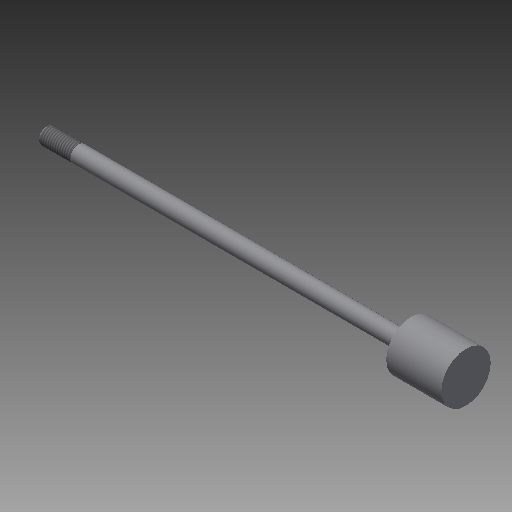
# Autodesk Inventor part: 043.5-DXP0000_rod
Saved by Autodesk Inventor 2019 (Build 230136000, 136)
## iProperties
Category: PARTsolutions
Company: BIMBA
Created: 2019-01-26
Part Number: 043.5-DXP0000_rod
Material: Generic
Catalog Web Link: www.cadenas.de
Description: Standard Air Cylinder_rod-Original Line - Standard Air Cylinders
Vendor: BIMBA
Document SubType Name: Modeling
Designer: psadmin
Manufacturer: BIMBA
Mass: 10.7288 g
Surface Area: 47.1446 cm^2
Volume: 10.7288 cm^3
Density: 1 g/cm^3
Appearance: PSOLRGB-181-181-181
PSOL_IDENT_0: {$CADENAS_DATA\23d-libs\bimba\bimba\bimba_imperial\bimba_full_line\original_line_cylinders\standard_
PSOL_IDENT_1: air_cylinders\rod.prj},327 {VTYP=3D},{NB=043.5-DXP0000_rod},{LINA=043.5-DXP0000_rod},{NN=Standard Ai
PSOL_IDENT_2: r Cylinder_rod},{DATE=21.03.2018 14:31:21},{GEOMDATE=09.11.2017 13:09:15},{VERSION=},{LINEID=50},{WB
PSOL_IDENT_3: VAR=STROKE,ACTING,MNT,DER,NR,BM,CO,M,EE,EEL,K,Q,Y,F,G,T,B,H,SER,SR,NT,W,E,HL,ST,STP,PRC,PB,COLOR1,FC
PSOL_IDENT_4: D,RCD,BCD},{WBNUMERIC=STROKE,EEL,COLOR1,FCD,RCD,BCD}  {NB=043.5-DXP0000_rod},{LINA=043.5-DXP0000_rod
PSOL_IDENT_5: },{KT=DUMMY},{PN=043.5-DXP000},{DASH=-},{BORE=0.75000000},{BOREPN=04},{STROKE=3.500},{STROKEALG=[0.0
PSOL_IDENT_6: 01:50/0.001]},{STROKE1=3.500},{ACTING=D},{ACTINGALG= '' , 'Single Acting' , 'R' , 'Reverse Single Ac
PSOL_IDENT_7: ting' , 'D' , 'Double Acting' },{ACTINGPN=D},{MNT=XP},{MNTALG= '' , 'Front Nose Mounting' , 'P' , 'R
PSOL_IDENT_8: ear Pivot Mounting' , 'XP' , 'Double End or Pivot Mounting' , 'X' , 'Double End Mounting' , 'BF' , '
PSOL_IDENT_9: Front Block Mounting' , 'BR' , 'Rear Block Mounting for Vertical Positioning' , 'BFT' , 'Front Block
PSOL_IDENT_10: Trunnion Mounting' , 'BRT' , 'Rear Block Trunnion Mounting' },{TYPE=},{MNTPN=XP},{DER=},{DERALG= ''
PSOL_IDENT_11: , 'N/A' },{NR=},{NRALG= '' , 'N/A' },{NRPN=},{BM=},{BMALG= '' , 'N/A' },{BMPN=},{CO=},{COALG= '' , '
PSOL_IDENT_12: N/A' },{M=},{MALG= '', 'Without Magnet', 'M', 'With Magnet' },{EE=},{EEL=0},{EEMAX=46},{EEALG= '', '
PSOL_IDENT_13: Without Extra Extension', 'EE', 'With Extra Extension' },{EELALG=0},{EEPN=},{EEPN1=0.000},{K=},{KALG=
PSOL_IDENT_14: '', 'Standard' , 'K' , 'Ports Rotated 90deg' },{KPN=},{Q=},{QALG= '' , 'Without Side Ported Rear He
PSOL_IDENT_15: ad' , 'Q' , 'With Side Ported Rear Head' },{QPN=},{Y=},{YALG= '' , 'Without Pivot Bushing' , 'Y' , '
PSOL_IDENT_16: With Pivot Bushing' },{YPN=},{F=},{FALG= '', 'Standard', 'F', 'Molycoated Body' },{FPN=},{G=},{GPN=}
PSOL_IDENT_17: ,{T=},{TALG= '' , 'Standard' , 'N' , 'Low Temperature' , 'V' , 'High Temperature' },{NPN=},{VPN=},{B=
PSOL_IDENT_18: },{BALG= '', 'Without Bumper' , 'B' , 'With Bumper' },{BPN=},{H=},{HALG= '', 'N/A' },{HPN=},{SER=},{
PSOL_IDENT_19: SERALG= '' , 'Without Spring Extend/Return' , 'JS' , 'With Spring Return' , 'JR' , 'With Spring Exte
PSOL_IDENT_20: nd' },{SR=},{SRALG= 'C' , 'Carbon Steel Rod' , 'SR' , '303 Stainless Steel Rod' , '' , '303 Stainles
PSOL_IDENT_21: s Steel Rod1' },{SRPN=},{SRCON=0},{NT=},{NTPN=},{W=},{WALG= '' , 'Without Wiper' , 'W' , 'With Wiper'
PSOL_IDENT_22: },{WPN=},{E=},{EALG= '' , 'Without Special Lube and Seals' , 'E' , 'With Special Lube and Seals' },
PSOL_IDENT_23: {EPN=},{HL=},{HLALG= '' , 'Wihout Low Pressure Hydraulic' , 'HL' , 'With Low Pressure Hydraulic' },{
PSOL_IDENT_24: ST=},{STALG= '' , 'Without Switch Track' , 'T' , 'With Switch Track' },{STP=},{STPALG= '' , 'N/A' },
PSOL_IDENT_25: {STPN=},{PRC=},{PRCALG= '' , 'Without Piston Rod Clevis' , 'D-166-1' , 'With Piston Rod Clevis' },{P
PSOL_IDENT_26: RCPN=},{PB=},{PBALG= '' , 'Without Pivot Bracket' , 'D-167' , 'With Pivot Bracket' },{PBPN=},{TLEN=4
PSOL_IDENT_27: .7555},{TEXT=0.333333},{SPACE=0.190476},{FRAC=17.2500},{RGCON=},{RGDACCON=R},{RHCON=P},{RHCONON=1},{
PSOL_IDENT_28: RHACCON=},{FNUTCON=1},{RNUTCON=1},{FNUTPN=D-9},{RNUTPN=D-9},{FNUTTRANS=0.0000},{RNUTTRANS=0.0000},{V
PSOL_IDENT_29: HOLECON=0},{A1=1.5940},{A1N=0.8750},{A1P=1.5940},{A1B=1.5940},{A4=0.2525},{A4N=0.3130},{A4P=0.2525},
PSOL_IDENT_30: {A5=0.0300},{A1H=1.594},{A1NH=0.5310},{A1PH=1.5940},{A1BH=1.0940},{A1SH=1.2190},{A2H=0.2190},{A2NH=0
PSOL_IDENT_31: .2190},{LENGTH=3.7500},{LENGTH1=3.7500},{LENGTH2=3.8100},{MUL=3.5000},{MUL11=3.5000},{MUL22=9.4150},
PSOL_IDENT_32: {MUL33=5.9150},{MUL2=3.5000},{MUL211=3.5000},{MUL222=2.6900},{MUL233=1.6900},{SSS=7.0000},{RGLEN=1.3
PSOL_IDENT_33: 715},{RHLEN=1.1230},{SSS1=4.0000},{A13=1.3120},{THDLEN1=0.5000},{THD1=0.2500},{TAB=UNF},{THDLEN=0.50
PSOL_IDENT_34: 00},{THD=0.2500},{OD=0.7615},{RODL=6.4380},{PL=0.8440},{RODDIA=0.2500},{HEX=0.2500},{RODTRANS=0.0000
PSOL_IDENT_35: },{G1=0.1250},{ON=0},{G5=0.6250},{DERLEN=5.5940},{THOLE=0.0000},{WF=0.2200},{BADD=0.0000},{MADD=0.00
PSOL_IDENT_36: 00},{NVADD=0.000},{JRADD=0.00000},{COLOR=0.71,0.71,0.71,0.00},{GROOVE=1},{HOL=1},{D7=0.2520},{H1=1.1
PSOL_IDENT_37: 175},{D1=0.8625},{D1RH=0.8625},{D1P=0.8325},{D1B=0.8625},{D1N=0.8050},{D1NRH=0.8050},{D1BRH=0.8325},
PSOL_IDENT_38: {D1PRH=0.8625},{BOZO=0},{HADD=0.000},{COLOR1=0},{DEFL=0.0000},{HEXL=0.0000},{SSADD=0.0000},{WFL=0.00
PSOL_IDENT_39: 00},{MOVE=0.0000},{PRCL2=0.50000},{PRCB=0.16000},{PRCTRANS=0.16000},{FCD=0},{RCD=0},{BCD=0}
NN: Standard Air Cylinder_rod
NT: Standard
NB: 043.5-DXP0000_rod
NBSYN: $PN.$COLOR1._rod
LINA: 043.5-DXP0000_rod
PN: 043.5-DXP000
BORE: 0.75
BOREPN: 04
STROKE: 3.5
ACTING: Double Acting
MNT: Double End or Pivot Mounting
DER: N/A
NR: N/A
BM: N/A
CO: N/A
M: Without Magnet
EE: Without Extra Extension
EEL: 0
K: Standard
Q: Without Side Ported Rear Head
Y: Without Pivot Bushing
F: Standard
G: Without Magnalube Lubrication
T: Standard
B: Without Bumper
H: N/A
SER: Without Spring Extend/Return
SR: 303 Stainless Steel Rod1
W: Without Wiper
E: Without Special Lube and Seals
HL: Wihout Low Pressure Hydraulic
ST: Without Switch Track
STP: N/A
PRC: Without Piston Rod Clevis
PB: Without Pivot Bracket
A1N: 0.875
A1P: 1.594
A1B: 1.594
A4N: 0.313
A4P: 0.2525
A5: 0.03
A1NH: 0.531
A1PH: 1.594
A1BH: 1.094
A1SH: 1.219
A2NH: 0.219
A13: 1.312
THDLEN1: 0.5
THD1: 0.25
TAB: UNF
OD: 0.7615
RODDIA: 0.25
HEX: 0.25
G1: 0.125
G5: 0.625
THOLE: 0
WF: 0.22
GROOVE: 1
D7: 0.252
D1P: 0.8325
D1B: 0.8625
D1N: 0.805
D1NRH: 0.805
D1BRH: 0.8325
D1PRH: 0.8625
COLOR1: 0
FCD: 0
RCD: 0
BCD: 0
SUPPLIER: BIMBA
ARTICLENO: 043.5-DXP0000_rod
BOMINFO: 043.5-DXP0000_rod
CREATOR: CADENAS GmbH
Title: 043.5-DXP0000_rod
Author: Cadenas PARTsolutions
Comments: Original Line - Standard Air Cylinders
Autodesk Inventor part; units mm, degrees
ref_plane "YZ Plane" through (0, 0, 0) normal (1, 0, 0) x (0, 1, 0)
ref_plane "XZ Plane" through (0, 0, 0) normal (0, 1, 0) x (-1, 0, 0)
ref_plane "XY Plane" through (0, 0, 0) normal (0, 0, 1) x (1, 0, 0)
sketch "Sketch_1" plane through (0, 0, 0) normal (0, 0, 1) x (1, 0, 0)
  line L0 (150.8252, 0) -> (0, 0)
  line L1 (0, 0) -> (0, 3.175)
  line L2 (0, 3.175) -> (129.3876, 3.175)
  line L3 (129.3876, 3.175) -> (129.3876, 9.6203)
  line L4 (129.3876, 9.6203) -> (150.8252, 9.6203)
  line L5 (150.8252, 9.6203) -> (150.8252, 0)
  line L6 (150.8252, 0) -> (0, 0)
  constraints: 14 end point
revolve "Revolution1" add sketch "Sketch_1" angle 360 about axis through (150.8252, 0, 0) along (1, 0, 0)
sketch "Sketch_3" plane through (0, 0, 0) normal (0, 0, 1) x (1, 0, 0)
  line L0 (0, 0) -> (-12.7, 0)
  line L1 (-12.7, 0) -> (-12.7, 2.634)
  line L2 (-12.7, 2.634) -> (-12.159, 3.175)
  line L3 (-12.159, 3.175) -> (0, 3.175)
  line L4 (0, 3.175) -> (0, 0)
  line L5 (0, 0) -> (-12.7, 0)
  constraints: 12 end point
revolve "Revolution2" add sketch "Sketch_3" angle 360 about axis through (0, 0, 0) along (1, 0, 0)
thread "Thread1" size "1/4-28 UNF" class "2A" standard "ANSI Unified Screw Threads" length 12.159
sketch "Sketch_30" plane through (0, 0, 0) normal (0, 0, 1) x (1, 0, 0)
  line L0 (0, 0) -> (-0.254, 0)
  line L1 (-0.254, 2.921) -> (0, 2.921)
  line L2 (0, 2.921) -> (0, 3.429)
  line L3 (0, 3.429) -> (-0.254, 3.429)
  line L4 (-0.254, 3.429) -> (-0.254, 2.921)
  constraints: 10 end point
revolve "Revolution3" cut sketch "Sketch_30" angle 360 about axis through (0, 0, 0) along (1, 0, 0)
ref_plane "dia1_XY" through (0, 3.175, 0) normal (1, 0, 0) x (0, 0, -1)
ref_plane "dia1_YZ" through (0, 3.175, 0) normal (0, 0, -1) x (0, 1, 0)
ref_plane "dia1_ZX" through (0, 3.175, 0) normal (0, 1, 0) x (1, 0, 0)
ref_plane "dia12_XY" through (0, 0, 10.9537) normal (1, 0, 0) x (0, 0, -1)
ref_plane "dia12_YZ" through (0, 0, 10.9537) normal (0, 0, -1) x (0, 1, 0)
ref_plane "dia12_ZX" through (0, 0, 10.9537) normal (0, 1, 0) x (1, 0, 0)
ref_plane "dia2_XY" through (0, -3.175, 0) normal (1, 0, 0) x (0, 0, -1)
ref_plane "dia2_YZ" through (0, -3.175, 0) normal (0, 0, -1) x (0, 1, 0)
ref_plane "dia2_ZX" through (0, -3.175, 0) normal (0, 1, 0) x (1, 0, 0)
ref_plane "dia22_XY" through (0, 0, -10.9537) normal (1, 0, 0) x (0, 0, -1)
ref_plane "dia22_YZ" through (0, 0, -10.9537) normal (0, 0, -1) x (0, 1, 0)
ref_plane "dia22_ZX" through (0, 0, -10.9537) normal (0, 1, 0) x (1, 0, 0)
ref_plane "hh1_XY" through (180.9496, 0, 0) normal (0, 0, 1) x (1, 0, 0)
ref_plane "hh1_YZ" through (180.9496, 0, 0) normal (1, 0, 0) x (0, 1, 0)
ref_plane "hh1_ZX" through (180.9496, 0, 0) normal (0, 1, 0) x (0, 0, 1)
ref_plane "hh2_XY" through (187.3504, 0, 0) normal (0, 0, 1) x (1, 0, 0)
ref_plane "hh2_YZ" through (187.3504, 0, 0) normal (1, 0, 0) x (0, 1, 0)
ref_plane "hh2_ZX" through (187.3504, 0, 0) normal (0, 1, 0) x (0, 0, 1)
ref_plane "rl1_XY" through (-12.7, 0, 0) normal (1, 0, 0) x (0, 0, -1)
ref_plane "rl1_YZ" through (-12.7, 0, 0) normal (0, 0, -1) x (0, 1, 0)
ref_plane "rl1_ZX" through (-12.7, 0, 0) normal (0, 1, 0) x (1, 0, 0)
ref_plane "rl2_XY" through (0, 0, 0) normal (1, 0, 0) x (0, 0, -1)
ref_plane "rl2_YZ" through (0, 0, 0) normal (0, 0, -1) x (0, 1, 0)
ref_plane "rl2_ZX" through (0, 0, 0) normal (0, 1, 0) x (1, 0, 0)
ref_plane "rod_cp_XY" through (0, 0, 0) normal (1, 0, 0) x (0, 0, -1)
ref_plane "rod_cp_YZ" through (0, 0, 0) normal (0, 0, -1) x (0, 1, 0)
ref_plane "rod_cp_ZX" through (0, 0, 0) normal (0, 1, 0) x (1, 0, 0)
ref_plane "thd1_XY" through (-12.7, 3.175, 0) normal (1, 0, 0) x (0, 0, -1)
ref_plane "thd1_YZ" through (-12.7, 3.175, 0) normal (0, 0, -1) x (0, 1, 0)
ref_plane "thd1_ZX" through (-12.7, 3.175, 0) normal (0, 1, 0) x (1, 0, 0)
ref_plane "thd2_XY" through (-12.7, -3.175, 0) normal (1, 0, 0) x (0, 0, -1)
ref_plane "thd2_YZ" through (-12.7, -3.175, 0) normal (0, 0, -1) x (0, 1, 0)
ref_plane "thd2_ZX" through (-12.7, -3.175, 0) normal (0, 1, 0) x (1, 0, 0)
ref_plane "to_rod_clevis_XY" through (-16.764, 0, 0) normal (1, 0, 0) x (0, 0, -1)
ref_plane "to_rod_clevis_YZ" through (-16.764, 0, 0) normal (0, 0, -1) x (0, 1, 0)
ref_plane "to_rod_clevis_ZX" through (-16.764, 0, 0) normal (0, 1, 0) x (1, 0, 0)
body "Solid1"
